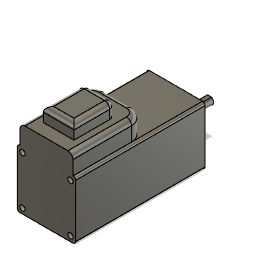
Mouting Plate BOB v13 (Autodesk Fusion 360 archive; units mm, degrees)
design "NEMA 23 Integrated Easy Servo Motor 130w"
Autodesk Fusion 360 part; units mm, degrees
sketch "Sketch1" plane through (0, 0, 0) normal (0, 0, 1) x (1, 0, 0)
  line L0 (0, 0) -> (57.15, 0)
  line L1 (57.15, 0) -> (57.15, 57.15)
  line L2 (57.15, 57.15) -> (0, 57.15)
  line L3 (0, 57.15) -> (0, 0)
  circle A0 centre (52.125, 52.125) radius 2.6
  line L4 (28.575, 0) -> (28.575, 57.15) construction
  line L5 (0, 28.575) -> (57.15, 28.575) construction
  circle A1 centre (5.025, 52.125) radius 2.6
  circle A2 centre (5.025, 5.025) radius 2.6
  circle A3 centre (52.125, 5.025) radius 2.6
  circle A4 centre (28.575, 28.575) radius 19.05
  line L6 (2.575, 57.15) -> (54.575, 57.15)
  line L7 (54.575, 57.15) -> (54.575, 76)
  line L8 (54.575, 76) -> (2.575, 76)
  line L9 (2.575, 76) -> (2.575, 57.15)
  circle A5 centre (28.575, 28.575) radius 4
  line L10 (26.6385, 32.075) -> (30.5115, 32.075)
  line L11 (13.575, 76) -> (43.575, 76)
  line L12 (43.575, 76) -> (43.575, 89.67)
  line L13 (43.575, 89.67) -> (13.575, 89.67)
  line L14 (13.575, 89.67) -> (13.575, 76)
  point P0 (47.5479, 45.3005)
  dimension "d1" = 57.15
  dimension "d2" = 57.15
  dimension "d3" = 5.2
  dimension "d5" = 5.2
  dimension "d6" = 47.1
  dimension "d8" = 5.2
  dimension "d10" = 47.1
  dimension "d12" = 5.2
  dimension "d13" = 47.1
  dimension "d14" = 47.1
  dimension "d15" = 38.1
  dimension "d16" = 76
  dimension "d17" = 8
  dimension "d19" = 3.5
  dimension "d20" = 52
  dimension "d21" = 13.67
  dimension "d22" = 30
  constraint horizontal L0
  constraint vertical L1
  constraint horizontal L2
  constraint vertical L3
  constraint coincident L0.start L3.end
  constraint midpoint L0 L4.start
  constraint midpoint L2 L4.end
  constraint midpoint L3 L5.start
  constraint midpoint L1 L5.end
  constraint symmetric A0 L4 A1
  constraint symmetric L5 A1.centre A2.centre
  constraint midpoint L5 A4.centre
  constraint horizontal L6
  constraint vertical L7
  constraint horizontal L8
  constraint vertical L9
  constraint coincident L2 L6.start
  constraint concentric A4 A5
  constraint coincident A5 L10.start
  constraint coincident A5 L10.end
  constraint perpendicular L4 L10
  constraint symmetric L4 L7 L9
  constraint horizontal L11
  constraint vertical L12
  constraint horizontal L13
  constraint vertical L14
  constraint coincident L8 L11.start
  constraint symmetric L4 L12 L14
  measures "d1" distance of L0.start L0.end
  measures "d2" distance of L0.start L2.end
  measures "d3" diameter of A0
  measures "d5" diameter of A1
  measures "d6" distance of A0.centre A1.centre
  measures "d8" diameter of A2
  measures "d10" distance of A1.centre A2.centre
  measures "d12" diameter of A3
  measures "d13" horizontal distance of A2.centre A3.centre
  measures "d14" distance of A0.centre A3.centre
  measures "d15" diameter of A4
  measures "d16" distance of L0 L8
  measures "d17" diameter of A5
  measures "d19" distance of L5 L10
  measures "d20" distance of L7.end L8.end
  measures "d21" distance of L11.start L13.end
  measures "d22" distance of L12.end L13.end
extrude "Extrude1" add sketch "Sketch1" along normal blind 127 contours L0 L1 L2 L3 L6 | A4 | A5 L10 | A5 L10
fillet "Fillet1" radius 2.5 4 edges at (57.15, 57.15, 63.5) (57.15, 0, 63.5) (0, 0, 63.5) (0, 57.15, 63.5)
extrude "Extrude2" add sketch "Sketch1" against normal blind 70 from surface at 127 contours L2 L6 L7 L8 L9 L11
fillet "Fillet2" radius 12.5 2 edges at (54.575, 66.575, 57) (2.575, 66.575, 57)
fillet "Fillet2" radius 5 3 edges at (54.575, 76, 92) (28.575, 76, 57) (2.575, 76, 92)
extrude "Extrude3" add sketch "Sketch1" along normal blind 40 from surface at 75 contours L8 L11 L12 L13 L14
fillet "Fillet3" radius 5 6 edges at (43.575, 89.67, 95) (43.575, 82.835, 75) (13.575, 82.835, 75) (28.575, 89.67, 75) (13.575, 89.67, 95) (28.575, 89.67, 115)
extrude "Extrude4" add sketch "Sketch1" against normal blind 2 contours A4 | A5 L10 | A5 L10
extrude "Extrude5" add sketch "Sketch1" against normal blind 33 contours A5 L10 picked at (29.5161, 29.5962)
extrude "Extrude6" add sketch "Sketch1" against normal blind 6 contours A5 L10 picked at (28.1041, 32.1557)
equation "d10 = d6"
equation "d12 = d3"
equation "d13 = d6"
equation "d14 = d6"
equation "d19 = 7.5 mm - ( d17 / 2 )"
equation "d44 = ( -1 * ( 33 - 27 ) ) * 1 mm"

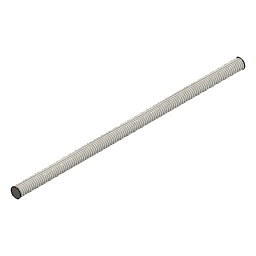
design "8mm T8 Lead Screw (190mm) v1"
Autodesk Fusion 360 part; units mm, degrees
sketch "Sketch1" plane through (0, 0, 0) normal (0, 0, 1) x (1, 0, 0)
  circle A0 centre (0, 0) radius 4
  dimension "d1" = 8
  constraint coincident A0.centre origin
  measures "d1" diameter of A0
extrude "Extrude1" add sketch "Sketch1" along normal blind 190
thread "Thread1" "ISO Metric Trapezoidal Threads 8.0 TR8x1.5 7e" major diameter 7.925 minor diameter 6.0605 pitch 1.5 angle 30 resizes the face on face at (3.995, -0.1994, 126.6667)

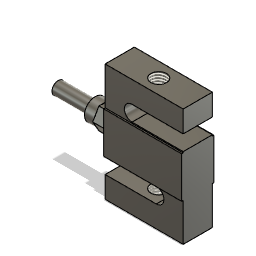
design "Load Cell (300 kg) v1"
Autodesk Fusion 360 part; units mm, degrees
sketch "Sketch1" plane through (0, 0, 0) normal (0, 0, 1) x (1, 0, 0)
  line L0 (0, 0) -> (50.75, 0)
  line L1 (50.75, 0) -> (50.75, 52.25)
  line L2 (50.75, 52.25) -> (12.5, 52.25)
  line L3 (12.5, 52.25) -> (12.5, 62.25)
  line L4 (12.5, 62.25) -> (50.75, 62.25)
  line L5 (50.75, 62.25) -> (50.75, 76.25)
  line L6 (50.75, 76.25) -> (0, 76.25)
  line L7 (0, 76.25) -> (0, 24)
  line L8 (0, 24) -> (38.25, 24)
  line L9 (38.25, 24) -> (38.25, 14)
  line L10 (38.25, 14) -> (0, 14)
  line L11 (0, 14) -> (0, 0)
  line L12 (0, 24.75) -> (50.75, 24.75)
  line L13 (50.75, 51.5) -> (0, 51.5)
  dimension "d1" = 76.25
  dimension "d2" = 14
  dimension "d3" = 10
  dimension "d4" = 50.75
  dimension "d5" = 12.5
  dimension "d6" = 0.75
  dimension "d7" = 0.75
  constraint coincident L0.start L11.end
  constraint horizontal L0
  constraint perpendicular L0 L1
  constraint perpendicular L1 L2
  constraint perpendicular L2 L3
  constraint perpendicular L3 L4
  constraint perpendicular L4 L5
  constraint perpendicular L5 L6
  constraint perpendicular L6 L7
  constraint perpendicular L7 L8
  constraint perpendicular L8 L9
  constraint perpendicular L9 L10
  constraint perpendicular L0 L11
  constraint equal L5 L11
  constraint equal L3 L9
  constraint collinear L7 L11
  constraint collinear L1 L5
  constraint equal L2 L10
  constraint coincident L7 L12.start
  constraint coincident L1 L12.end
  constraint perpendicular L1 L12
  constraint coincident L1 L13.start
  constraint coincident L7 L13.end
  constraint perpendicular L7 L13
  measures "d1" distance of L0 L6
  measures "d2" distance of L4.end L5.end
  measures "d3" distance of L2.end L3.end
  measures "d4" distance of L5.end L6.end
  measures "d5" distance of L1 L9
  measures "d6" distance of L8 L12
  measures "d7" distance of L2 L13
extrude "Extrude1" add sketch "Sketch1" along normal mid plane 19
extrude "Extrude2" add sketch "Sketch1" along normal mid plane 21 contours L1 L7 L12 L13
sketch "Sketch2" plane through (0, 0, 0) normal (-1, 0, 0) x (0, 0, 1)
  line L0 (9.5, 51.5) -> (9.5, 76.25)
  line L1 (9.5, 76.25) -> (-9.5, 76.25)
  line L2 (-9.5, 76.25) -> (-9.5, 51.5)
  line L3 (-9.5, 51.5) -> (-10.5, 51.5)
  line L4 (-10.5, 51.5) -> (-10.5, 24.75)
  line L5 (-10.5, 24.75) -> (-9.5, 24.75)
  line L6 (-9.5, 24.75) -> (-9.5, 24)
  line L7 (-9.5, 24) -> (9.5, 24)
  line L8 (9.5, 24) -> (9.5, 24.75)
  line L9 (9.5, 24.75) -> (10.5, 24.75)
  line L10 (10.5, 24.75) -> (10.5, 51.5)
  line L11 (10.5, 51.5) -> (9.5, 51.5)
  line L12 (8.0829, 38.125) -> (4.0415, 45.125)
  line L13 (4.0415, 45.125) -> (-4.0415, 45.125)
  line L14 (-4.0415, 45.125) -> (-8.0829, 38.125)
  line L15 (-8.0829, 38.125) -> (-4.0415, 31.125)
  line L16 (-4.0415, 31.125) -> (4.0415, 31.125)
  line L17 (4.0415, 31.125) -> (8.0829, 38.125)
  line L18 (-9.5, 0) -> (9.5, 0)
  line L19 (0, 76.25) -> (0, 24)
  circle A0 centre (0, 38.125) radius 4.1
  circle A1 centre (0, 38.125) radius 7
  point P0 (0, 38.125)
  dimension "d12" = 7
  dimension "d13" = 38.125
  dimension "d14" = 8.2
  dimension "d15" = 14
  constraint horizontal L16
  constraint coincident P0 L19
  constraint coincident P0 A0.centre
  constraint concentric A0 A1
  measures "d12" distance of P0 L17
  measures "d13" distance of P0 L18
  measures "d14" diameter of A0
  measures "d15" diameter of A1
extrude "Extrude3" add sketch "Sketch2" along normal blind 9.5 contours L13 L14 A1 | L19 A0 A1 | L12 L13 A1 | L19 A0 A1 | L19 A0 | L19 A0 | L12 L17 A1 | L14 L15 A1 | L15 L16 A1 | L16 L17 A1
extrude "Extrude4" add sketch "Sketch2" along normal blind 16 contours L19 A0 A1 | L19 A0 A1 | L19 A0 | L19 A0
extrude "Extrude5" add sketch "Sketch2" along normal blind 40 contours L19 A0 | L19 A0
fillet "Fillet1" radius 5 4 edges at (38.25, 14, 0) (38.25, 24, 0) (12.5, 62.25, 0) (12.5, 52.25, 0)
sketch "Sketch3" plane through (0, 76.25, 0) normal (0, 1, 0) x (-1, 0, 0)
  line L0 (0, -9.5) -> (0, 9.5)
  line L1 (0, 9.5) -> (-50.75, 9.5)
  line L2 (-50.75, 9.5) -> (-50.75, -9.5)
  line L3 (-50.75, -9.5) -> (0, -9.5)
  circle A0 centre (-25.375, 0) radius 6
  line L4 (0, 4.0415) -> (0, -4.0415)
  line L5 (-50.75, 0) -> (0, 0)
  dimension "d24" = 25.375
  dimension "d25" = 12
  constraint coincident A0.centre L5
  measures "d24" distance of A0.centre L4
  measures "d25" diameter of A0
extrude "Extrude6" cut sketch "Sketch3" against normal up to surface (14 mm away) contours A0 L5 | A0 L5
extrude "Extrude7" cut sketch "Sketch3" along normal up to surface (14 mm away) from surface at -76.25 contours A0 L5 | A0 L5
thread "Thread1" "ISO Metric profile 12.0 M12x1.75 6H" major diameter 12.2265 minor diameter 10.2735 pitch 1.75 angle 60 resizes the face on face at (19.3825, 66.9167, -0.2991)
thread "Thread2" "ISO Metric profile 12.0 M12x1.75 6H" major diameter 12.2265 minor diameter 10.2735 pitch 1.75 angle 60 resizes the face on face at (19.4048, 4.6667, -0.5974)
equation "d8 = ( 19 / 2 ) * 1 mm"
equation "d10 = ( 21 / 2 ) * 1 mm"
equation "d12 = ( 14 / 2 ) * 1 mm"
equation "d13 = d1 / 2"
equation "d24 = d4 / 2"

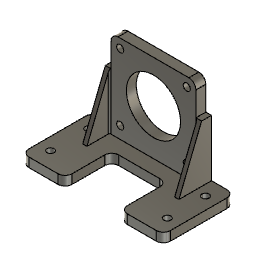
design "Soporte Nema"
Autodesk Fusion 360 part; units mm, degrees
sketch "Boceto2" plane through (0, 0, 0) normal (0, 0, 1) x (1, 0, 0)
  line L0 (0, 0) -> (100, 0)
  line L1 (100, 0) -> (100, 50)
  line L2 (100, 50) -> (0, 50)
  line L3 (0, 50) -> (0, 0)
  dimension "d5" = 100
  dimension "d6" = 50
  constraint horizontal L0
  constraint vertical L1
  constraint horizontal L2
  constraint vertical L3
  constraint coincident L0.start L3.end
  measures "d5" distance of L0.start L0.end
  measures "d6" distance of L0.start L2.end
extrude "Extruir2" add sketch "Boceto2" along normal blind 6.5
sketch "Boceto4" plane through (0, 0, 6.5) normal (0, 0, 1) x (-1, 0, 0)
  line L0 (0, -50) -> (0, 0)
  line L1 (0, 0) -> (-100, 0)
  line L2 (-100, 0) -> (-100, -50)
  line L3 (-100, -50) -> (0, -50)
  line L4 (0, -50) -> (-100, 0) construction
  line L5 (-100, -50) -> (0, 0) construction
  line L6 (-91.25, -38.5) -> (-8.75, -38.5) construction
  line L7 (-8.75, -38.5) -> (-8.75, -11.5) construction
  line L8 (-8.75, -11.5) -> (-91.25, -11.5) construction
  line L9 (-91.25, -11.5) -> (-91.25, -38.5) construction
  circle A0 centre (-8.75, -38.5) radius 2.5
  circle A1 centre (-91.25, -38.5) radius 2.5
  circle A2 centre (-91.25, -11.5) radius 2.5
  circle A3 centre (-8.75, -11.5) radius 2.5
  line L10 (-50, -25) -> (-50, 0) construction
  line L11 (-30.5, 33) -> (-69.5, 33)
  line L12 (-69.5, 33) -> (-69.5, -33)
  line L13 (-69.5, -33) -> (-30.5, -33)
  line L14 (-30.5, -33) -> (-30.5, 33)
  line L15 (-16, -50) -> (-19, -50)
  line L16 (-19, -43) -> (-19, -27)
  line L17 (-19, -27) -> (-16, -27)
  line L18 (-16, -27) -> (-16, -50)
  line L19 (-81, -43) -> (-81, -27)
  line L20 (-84, -50) -> (-81, -50)
  line L21 (-84, -27) -> (-84, -50)
  line L22 (-81, -27) -> (-84, -27)
  line L23 (-81, -50) -> (-80, -50)
  line L24 (-80, -50) -> (-80, -43)
  line L25 (-80, -43) -> (-81, -43)
  line L26 (-19, -50) -> (-20, -50)
  line L27 (-20, -50) -> (-20, -43)
  line L28 (-20, -43) -> (-19, -43)
  point P0 (-50, -25)
  point P1 (-50, 0)
  dimension "d11" = 82.5
  dimension "d12" = 27
  dimension "d13" = 5
  dimension "d18" = 39
  dimension "d19" = 66
  dimension "d31" = 27
  dimension "d32" = 3
  dimension "d33" = 31
  dimension "d36" = 1
  dimension "d37" = 7
  dimension "d38" = 1
  dimension "d39" = 7
  constraint coincident L0.start L3.end
  constraint coincident L1.end L2.start
  constraint coincident L2.end L3.start
  constraint coincident L0.end L1.start
  constraint horizontal L6
  constraint perpendicular L6 L7
  constraint parallel L6 L8
  constraint parallel L7 L9
  constraint midpoint L5 P0
  constraint coincident L6.end L7.start
  constraint coincident L6.start L9.end
  constraint coincident L8.end L9.start
  constraint coincident L7.end L8.start
  constraint equal A0 A3
  constraint equal A0 A2
  constraint equal A0 A1
  constraint coincident P0 L10.start
  constraint midpoint L1 P1
  constraint horizontal L11
  constraint perpendicular L11 L12
  constraint parallel L11 L13
  constraint parallel L12 L14
  constraint coincident P1 L10.end
  constraint horizontal L15
  constraint vertical L16
  constraint horizontal L17
  constraint vertical L18
  constraint coincident L3 L15.start
  constraint symmetric L10 L15.start L20.start
  constraint symmetric L10 L15.end L20.end
  constraint symmetric L10 L16.end L19.end
  constraint symmetric L10 L17.end L21.start
  constraint horizontal L23
  constraint vertical L24
  constraint horizontal L25
  constraint horizontal L26
  constraint vertical L27
  constraint horizontal L28
  measures "d11" distance of L7.end L8.end
  measures "d12" distance of L6.end L7.end
  measures "d13" diameter of A0
  measures "d18" distance of L12.end L13.end
  measures "d19" distance of L11.end L12.end
  measures "d31" distance of L1 L17
  measures "d32" distance of L16.end L17.end
  measures "d33" distance of L10 L16
  measures "d36" distance of L20.end L23.end
  measures "d37" distance of L20.end L19.start
  measures "d38" distance of L15.end L26.end
  measures "d39" distance of L15.end L16.start
extrude "Extruir3" cut sketch "Boceto4" against normal blind 20 contours L1 L12 L13 L14 | L1 L11 L12 L14 | A0 | A1 | A2 | A3
sketch "Boceto5" plane through (0, 50, 0) normal (0, 1, 0) x (-1, 0, 0)
  line L0 (0, 6.5) -> (-100, 6.5)
  line L1 (-100, 0) -> (0, 0)
  line L2 (-50, 6.5) -> (-50, 38.55) construction
  line L3 (-26.45, 15) -> (-73.55, 15) construction
  line L4 (-73.55, 15) -> (-73.55, 62.1) construction
  line L5 (-73.55, 62.1) -> (-26.45, 62.1) construction
  line L6 (-26.45, 62.1) -> (-26.45, 15) construction
  circle A0 centre (-73.55, 15) radius 2.5
  circle A1 centre (-26.45, 15) radius 2.5
  circle A2 centre (-26.45, 62.1) radius 2.5
  circle A3 centre (-73.55, 62.1) radius 2.5
  circle A4 centre (-50, 38.55) radius 19.15
  line L7 (-80, 6.5) -> (-20, 6.5)
  line L8 (-20, 6.5) -> (-20, 68.5)
  line L9 (-20, 68.5) -> (-80, 68.5)
  line L10 (-80, 68.5) -> (-80, 6.5)
  line L11 (-26.45, 62.1) -> (-73.55, 15) construction
  line L12 (-73.55, 62.1) -> (-26.45, 15) construction
  line L13 (0, 0) -> (0, 6.5)
  line L14 (-100, 6.5) -> (-100, 0)
  line L15 (0, 6.5) -> (-100, 6.5) construction
  line L16 (-69.5, 0) -> (-30.5, 0) construction
  point P0 (-50, 6.5)
  point P1 (-50, 38.55)
  point P2 (-50, 38.55)
  point P3 (-50, 38.55)
  point P4 (-100, 6.5)
  dimension "d27" = 47.1
  dimension "d28" = 47.1
  dimension "d29" = 5
  dimension "d30" = 38.3
  dimension "d44" = 60
  dimension "d45" = 62
  dimension "d48" = 15
  constraint midpoint L0 P0
  constraint perpendicular L0 L2
  constraint coincident P0 L2.start
  constraint horizontal L3
  constraint perpendicular L3 L4
  constraint parallel L3 L5
  constraint parallel L4 L6
  constraint coincident P3 P2
  constraint coincident L3.end L4.start
  constraint coincident L3.start L6.end
  constraint coincident L5.end L6.start
  constraint coincident L4.end L5.start
  constraint equal A0 A3
  constraint equal A0 A2
  constraint equal A0 A1
  constraint horizontal L7
  constraint perpendicular L7 L8
  constraint parallel L7 L9
  constraint parallel L8 L10
  constraint midpoint L11 P3
  constraint coincident L0.start L13.end
  constraint coincident P4 L0.end
  constraint coincident L7 P4
  measures "d27" distance of L4.end L5.end
  measures "d28" distance of L3.end L4.end
  measures "d29" diameter of A0
  measures "d30" diameter of A4
  measures "d44" distance of L8.end L9.end
  measures "d45" distance of L7.end L8.end
  measures "d48" distance of L3 L16
extrude "Extruir4" add sketch "Boceto5" against normal blind 7
extrude "Extruir5" add sketch "Boceto4" along normal blind 40 contours L3 L15 L16 L17 L18 L26 L27 L28 | L3 L19 L20 L21 L22 L23 L24 L25
chamfer "Chaflán1" distance 16 distance2 40 2 edges at (17.5, 27, 46.5) (82.5, 27, 46.5) measured on face at (18.3333, 47.6667, 46.5) measured on face at (81.6667, 47.6667, 46.5)
fillet "Empalme1" radius 5 4 edges at (0, 0, 3.25) (100, 0, 3.25) (100, 50, 3.25) (0, 50, 3.25)
fillet "Empalme1" radius 5 4 edges at (30.5, 0, 3.25) (30.5, 33, 3.25) (69.5, 0, 3.25) (69.5, 33, 3.25)
fillet "Empalme1" radius 5 2 edges at (80, 46.5, 68.5) (20, 46.5, 68.5)
fillet "Empalme2" radius 1 2 edges at (19, 43, 26.5) (81, 43, 26.5)

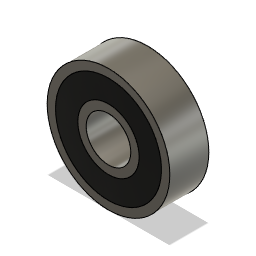
design "608 Bearings"
Autodesk Fusion 360 part; units mm, degrees
sketch "Sketch1" plane through (0, 0, 0) normal (0, 0, 1) x (1, 0, 0)
  circle A0 centre (0, 0) radius 11
  circle A1 centre (0, 0) radius 9.5
  circle A2 centre (0, 0) radius 4
  circle A3 centre (0, 0) radius 5.5
  dimension "d1" = 22
  dimension "d2" = -1.5
  dimension "d3" = 8
  dimension "d4" = 1.5
  constraint coincident A0.centre A1.centre
  measures "d1" diameter of A0
  measures "d3" diameter of A2
extrude "Extrude1" add sketch "Sketch1" along normal blind 7 makes body 1 at (5.4727, -0.5476, 4.6667) makes body 2 at (10.9453, -1.0952, 4.6667)
extrude "Extrude2" add sketch "Sketch1" along normal blind 7 separate body contours A1 makes body 3

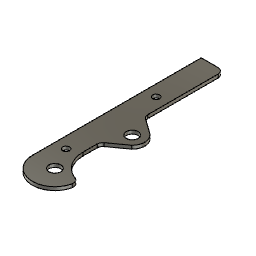
design "Pedal Inox"
Autodesk Fusion 360 part; units mm, degrees
sketch "Boceto1" plane through (0, 0, 0) normal (0, 0, 1) x (1, 0, 0)
  circle A0 centre (40, 0) radius 5.3
  line L0 (35, 150) -> (20, 150)
  arc A1 (56.3856, 1.531) -> (40, 25) centre (65, 25) cw
  line L1 (20, 20) -> (40.5051, 20)
  circle A2 centre (30, 20) radius 3
  line L2 (40, 0) -> (40, -27.0971) construction
  arc A3 (59.5504, -4.217) -> (56.3856, 1.531) centre (54.6628, -3.1628) ccw
  arc A4 (40, 145) -> (35, 150) centre (35, 145) ccw
  line L3 (20, 0) -> (20, 150)
  circle A5 centre (48.7119, 60) radius 5.3
  line L4 (42.0966, 78.4008) -> (54.9817, 69.2104)
  line L5 (42.0747, 41.5846) -> (56.3254, 51.8651)
  arc A6 (56.3254, 51.8651) -> (54.9817, 69.2104) centre (48.7119, 60) ccw
  arc A7 (40, 20) -> (40.5064, 19.9936) centre (40, 0) cw
  arc A8 (59.5504, -4.217) -> (20, 0) centre (40, 0) cw
  line L6 (40, 0) -> (40, 37.5296) construction
  line L7 (40, 60) -> (48.7119, 60) construction
  line L8 (40, 25) -> (40, 40.0879)
  line L9 (40, 82.4715) -> (40, 145)
  arc A9 (40, 82.4715) -> (42.0966, 78.4008) centre (45, 82.4715) ccw
  arc A10 (42.0747, 41.5846) -> (40, 37.5296) centre (45, 37.5296) ccw
  circle A11 centre (30, 100) radius 3
  point P0 (40, 22.5)
  point P1 (41.25, -20)
  point P2 (20, 150)
  dimension "d52" = 25
  dimension "d7" = 6
  dimension "d12" = 5
  dimension "d13" = 5
  dimension "d18" = 60
  dimension "d19" = 5
  dimension "d20" = 80
  constraint coincident P2 L0.end
  constraint tangent A1 A3
  constraint tangent L0 A4
  constraint coincident A1 L1.end
  constraint coincident L1 A2.centre
  constraint perpendicular L0 L3
  constraint equal A0 A5
  constraint coincident L1 A7.start
  constraint coincident A1 A7.end
  constraint concentric A7 A8
  constraint perpendicular L1 L6
  constraint perpendicular L7 L8
  constraint coincident A5.centre A6.centre
  constraint collinear L8 L9
  constraint tangent L9 A9
  constraint tangent L4 A9
  constraint coincident L5 L8.end
  constraint coincident L6 L8.end
  constraint tangent L5 A10
  constraint tangent L6 A10
  constraint equal A9 A10
  constraint equal A2 A11
  measures "d52" radius of A1
  measures "d7" diameter of A2
  measures "d12" radius of A3
  measures "d13" radius of A4
  measures "d18" distance of A0.centre L7.start
  measures "d19" radius of A9
  measures "d20" distance of A2.centre A11.centre
extrude "Extruir1" add sketch "Boceto1" along normal blind 3 contours L0 A1 L1 A2 A4 L3 L4 L5 A6 L8 L9 A9 A10 | A1 L1 A2 A3 L3 A7 A8 | A1 L1 A7

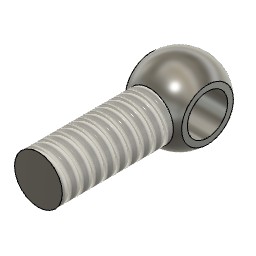
design "M12 Eye Screw (35mm)"
Autodesk Fusion 360 part; units mm, degrees
sketch "Sketch1" plane through (0, 0, 0) normal (0, 0, 1) x (1, 0, 0)
  circle A0 centre (0, 0) radius 6
  dimension "d1" = 12
  constraint coincident A0.centre origin
  measures "d1" diameter of A0
extrude "Extrude1" add sketch "Sketch1" along normal blind 30
thread "Thread1" "ISO Metric Trapezoidal Threads 12.0 TR12x3 7e" major diameter 11.882 minor diameter 8.3175 pitch 3 angle 30 resizes the face on face at (5.9702, -0.5974, 20)
extrude "Extruir2" add sketch "Sketch1" against normal blind 5
sketch "Boceto3" plane through (0, 0, 0) normal (1, 0, 0) x (0, 1, 0)
  line L0 (-6, -5) -> (6, -5) construction
  line L1 (-16.6983, -5) -> (23.2423, -5) construction
  circle A0 centre (0, -5) radius 5
  line L2 (-9.5, -5) -> (9.5, -5)
  arc A1 (-9.5, -5) -> (9.5, -5) centre (0, -5) ccw
  point P0 (0, -5)
  dimension "d8" = 10
  dimension "d9" = 19
  constraint parallel L0 L1
  constraint coincident P0 A0.centre
  constraint concentric A0 A1
  constraint coincident L1 L2.start
  constraint coincident L1 L2.end
  measures "d8" diameter of A0
  measures "d9" diameter of A1
revolve "Revolución1" add sketch "Boceto3" angle 360 about axis through (0, -16.6983, -5) along (0, 1, 0) contours A0 L2 A1 | A0 L2 picked at (0.1246, -6.662)
extrude "Extruir3" cut sketch "Boceto3" along normal blind -13 and the other way blind -20 contours A0 L2 | A0 L2
sketch "Boceto4" plane through (0, 0, 0) normal (0, 0, 1) x (1, 0, 0)
  line L0 (7, 12.157) -> (-7, 12.157)
  line L1 (-7, 12.157) -> (-7, -12.157)
  line L2 (-7, -12.157) -> (7, -12.157)
  line L3 (7, -12.157) -> (7, 12.157)
  line L4 (7, 12.157) -> (-7, -12.157) construction
  line L5 (-7, 12.157) -> (7, -12.157) construction
  line L6 (12.0025, 16.6058) -> (-12.0025, 16.6058)
  line L7 (-12.0025, 16.6058) -> (-12.0025, -16.6058)
  line L8 (-12.0025, -16.6058) -> (12.0025, -16.6058)
  line L9 (12.0025, -16.6058) -> (12.0025, 16.6058)
  line L10 (12.0025, 16.6058) -> (-12.0025, -16.6058) construction
  line L11 (-12.0025, 16.6058) -> (12.0025, -16.6058) construction
  dimension "d17" = 14
  constraint horizontal L0
  constraint perpendicular L0 L1
  constraint parallel L0 L2
  constraint parallel L1 L3
  constraint coincident L4 origin
  constraint coincident L5 origin
  constraint horizontal L6
  constraint perpendicular L6 L7
  constraint parallel L6 L8
  constraint parallel L7 L9
  constraint coincident L10 origin
  constraint coincident L11 origin
  measures "d17" distance of L0.start L0.end
extrude "Extruir4" cut sketch "Boceto4" along normal blind -105 and the other way blind -4

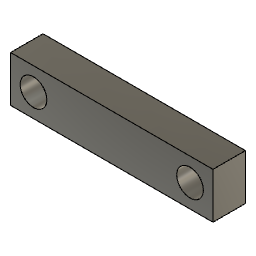
design "separador"
Autodesk Fusion 360 part; units mm, degrees
sketch "Boceto1" plane through (0, 0, 0) normal (0, 0, 1) x (1, 0, 0)
  line L0 (0, 0) -> (53, 0)
  line L1 (0, 0) -> (0, 8.5)
  line L2 (0, 8.5) -> (2.0137, 8.5)
  line L3 (2.0137, 8.5) -> (53, 8.5)
  line L4 (53, 8.5) -> (53, 0)
  dimension "d1" = 53
  dimension "d23" = 8.5
  constraint horizontal L0
  constraint coincident L0.start L1.start
  constraint perpendicular L0 L1
  constraint perpendicular L1 L2
  constraint parallel L0 L3
  constraint perpendicular L0 L4
  measures "d1" distance of L0.start L0.end
  measures "d23" distance of L0.start L1.end
extrude "Extruir1" add sketch "Boceto1" along normal blind 12
sketch "Boceto2" plane through (0, 8.5, 0) normal (0, 1, 0) x (-1, 0, 0)
  circle A0 centre (-6, 6) radius 3.5
  circle A1 centre (-47, 6) radius 3.5
  line L0 (-53, 0) -> (0, 0)
  line L1 (0, 12) -> (-53, 12)
  line L2 (-53, 12) -> (-53, 0)
  line L3 (-53, 0) -> (0, 0)
  line L4 (0, 0) -> (0, 12)
  line L5 (0, 12) -> (-53, 12)
  line L6 (-53, 12) -> (-53, 0)
  dimension "d13" = 7
  dimension "d15" = 6
  dimension "d16" = 7
  measures "d13" diameter of A0
  measures "d15" distance of A0.centre L1
  measures "d16" diameter of A1
extrude "Extruir2" cut sketch "Boceto2" against normal blind 25 contours A0 | A1

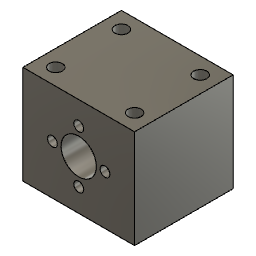
design "Lead Screw Nut Mount"
Autodesk Fusion 360 part; units mm, degrees
sketch "Sketch1" plane through (0, 0, 0) normal (0, 0, 1) x (1, 0, 0)
  circle A0 centre (0, 4) radius 5.375
  line L0 (-17, -11) -> (17, -11)
  line L1 (17, -11) -> (17, 19)
  line L2 (17, 19) -> (-17, 19)
  line L3 (-17, 19) -> (-17, -11)
  circle A1 centre (0, 12) radius 1.5
  circle A2 centre (-8, 4) radius 1.5
  circle A3 centre (0, -4) radius 1.5
  circle A4 centre (8, 4) radius 1.5
  dimension "d5" = 10.75
  dimension "d9" = 3
  dimension "d27" = 34
  dimension "d37" = 30
  constraint horizontal L0
  constraint vertical L1
  constraint horizontal L2
  constraint vertical L3
  measures "d5" diameter of A0
  measures "d9" diameter of A1
  measures "d27" distance of L1 L3
  measures "d37" distance of L0.end L1.end
extrude "Extrude1" add sketch "Sketch1" along normal blind 30
sketch "Sketch2" plane through (17, 0, 0) normal (1, 0, 0) x (0, 0, -1)
  line L0 (0, -11) -> (0, 19)
  line L1 (0, 19) -> (-30, 19)
  line L2 (-30, 19) -> (-30, -11)
  line L3 (-30, -11) -> (0, -11)
  circle A0 centre (-15, 44) radius 5
  line L4 (-15, 19) -> (-15, 44) construction
  circle A1 centre (-15, 44) radius 12.5
  line L5 (-30, 19) -> (-27.4409, 45.2145)
  line L6 (0, 19) -> (-2.5591, 45.2145)
  dimension "d20" = 10
  dimension "d35" = 25
  dimension "d36" = 25
  constraint midpoint L1 L4.start
  constraint perpendicular L1 L4
  constraint coincident A0.centre L4.end
  constraint concentric A0 A1
  constraint coincident L1.end L2.start
  constraint coincident A1 L5.end
  constraint tangent A1 L5
  constraint coincident L0.end L1.start
  constraint coincident A1 L6.end
  constraint tangent A1 L6
  measures "d20" diameter of A0
  measures "d35" distance of L4.start A0.centre
  measures "d36" diameter of A1
sketch "Boceto4" plane through (0, 19, 0) normal (0, 1, 0) x (-1, 0, 0)
  line L0 (-17, 0) -> (17, 0)
  line L1 (17, 0) -> (17, 30)
  line L2 (17, 30) -> (-17, 30)
  line L3 (-17, 30) -> (-17, 0)
  line L4 (-12, 25) -> (12, 25) construction
  line L5 (12, 25) -> (12, 5) construction
  line L6 (12, 5) -> (-12, 5) construction
  line L7 (-12, 5) -> (-12, 25) construction
  circle A0 centre (-12, 25) radius 2
  circle A1 centre (12, 25) radius 2
  circle A2 centre (12, 5) radius 2
  circle A3 centre (-12, 5) radius 2
  dimension "d40" = 24
  dimension "d41" = 20
  dimension "d42" = 5
  dimension "d43" = 5
  dimension "d44" = 4
  constraint horizontal L4
  constraint vertical L5
  constraint horizontal L6
  constraint vertical L7
  constraint coincident L4.start L7.end
  constraint coincident L4.end L5.start
  constraint coincident L5.end L6.start
  constraint coincident L6.end L7.start
  constraint equal A0 A3
  constraint equal A1 A3
  constraint equal A2 A3
  measures "d40" distance of L4.start L4.end
  measures "d41" distance of L4.end L5.end
  measures "d42" distance of L3 L7
  measures "d43" distance of L0 L6
  measures "d44" diameter of A3
extrude "Extruir4" cut sketch "Boceto4" against normal blind 4 contours A0 | A1 | A2 | A3
equation "Screw_Nut_Dia = 10 mm"
equation "Screw_Nut_bolt_Dia = 3 mm"
equation "Screw_Nut_Bolt_Pattern = 16 mm"
equation "d5 = Screw_Nut_Dia + 0.75 mm"
equation "d9 = Screw_Nut_bolt_Dia"
equation "d13 = Screw_Nut_bolt_Dia"
